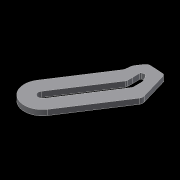
# Autodesk Inventor part: PelvisLinkLeft
Saved by Autodesk Inventor 2015 (Build 190159000, 159)
## iProperties
Created: 2014-12-04
Part Number: PelvisLinkLeft
Material: Generic
Document SubType Name: Modeling
Designer: Val
Density: 1 g/cm^3
Appearance: Default
Mass: 6.30084 g
Surface Area: 44.3973 cm^2
Volume: 6.30084 cm^3
Author: Val
Autodesk Inventor part; units mm, degrees
ref_plane "YZ Plane" through (0, 0, 0) normal (1, 0, 0) x (0, 1, 0)
ref_plane "XZ Plane" through (0, 0, 0) normal (0, 1, 0) x (-1, 0, 0)
ref_plane "XY Plane" through (0, 0, 0) normal (0, 0, 1) x (1, 0, 0)
sketch "Body" plane through (0, 0, 0) normal (0, 0, 1) x (1, 0, 0)
  line L0 (28.8487, 38.4543) -> (2.7256, -1.7701)
  line L1 (22.3487, 40.3798) -> (-2.7256, 1.7701)
  line L2 (22.3487, 40.3798) -> (22.3487, 45.0293)
  line L3 (28.8487, 38.4543) -> (28.8487, 45.9543)
  line L4 (32.4946, 58.4071) -> (39.19, 35.3599)
  line L5 (19.5232, 59.2689) -> (32.4946, 58.4071)
  line L6 (14.1445, 46.7648) -> (14.7577, 52.2305)
  line L7 (22.3487, 45.0293) -> (20.7935, 50.3829) construction
  line L8 (28.8487, 45.9543) -> (27.0354, 52.1963) construction
  arc A0 (-11.4127, 7.4118) -> (11.4127, -7.4118) centre (0, 0) ccw
  line L9 (-11.4127, 7.4118) -> (14.1445, 46.7648)
  line L10 (11.4127, -7.4118) -> (39.19, 35.3599)
  circle A1 centre (0, 0) radius 3.25
  line L11 (25.5987, 39.4171) -> (0, 0) construction
  line L12 (25.5987, 39.4171) -> (25.5987, 45.4918) construction
  line L13 (25.5987, 45.4918) -> (24.7618, 48.3727) construction
  line L14 (19.5232, 59.2689) -> (14.7577, 52.2305)
  line L15 (-30.4273, 0) -> (50.7929, 0) construction
  line L16 (20.7935, 50.3829) -> (22.2339, 50.8014) construction
  line L17 (22.3487, 45.0293) -> (22.2339, 50.8014)
  line L18 (28.8487, 45.9543) -> (25.595, 51.7778)
  line L19 (22.2339, 50.8014) -> (25.595, 51.7778)
  line L20 (25.595, 51.7778) -> (27.0354, 52.1963) construction
  dimension "d37" = 6.5
  dimension "d38" = 130.8
  dimension "d45" = 3.25
  dimension "d46" = 3.25
  dimension "d47" = 3.25
  dimension "d48" = 3.25
  dimension "d49" = 3.25
  dimension "d50" = 3.25
  dimension "d51" = 47
  dimension "d52" = 7.5
  dimension "d54" = 123.001
  dimension "d56" = 130.8
  dimension "d57" = 24
  dimension "d58" = 13
  dimension "d59" = 8.5
  dimension "d60" = 5.5
  dimension "d61" = 110
  dimension "d62" = 120.3
  dimension "d63" = 51
  dimension "d64" = 153.4
  dimension "d74" = 6.5
  dimension "d75" = 1.5
  dimension "d76" = 1.5
  constraints: 40 end point, 6 parallel, 4 point on circle, 3 perpendicular, 2 centre point, 2 tangent, 1 coincident, 1 point on line, 1 vertical
  measures "d37" diameter of A1
  measures "d38" angle of L11 L13
  measures "d45" distance between parallel lines of L1 L11
  measures "d46" distance between parallel lines of L2 L12
  measures "d47" distance between parallel lines of L7 L13
  measures "d48" distance between parallel lines of L0 L11
  measures "d49" distance between parallel lines of L3 L12
  measures "d50" distance between parallel lines of L13 L8
  measures "d51" distance of L11.end L11.start
  measures "d52" distance of L0.start L3.end
  measures "d54" angle of L9 L15
  measures "d56" angle of L10 L4
  measures "d57" distance of L4.start L4.end
  measures "d58" distance of L5.start L4.start
  measures "d59" distance of L5.start L6.end
  measures "d60" distance of L6.start L6.end
  measures "d61" angle of L4 L5
  measures "d62" angle of L5 L14
  measures "d63" distance of L10.start L4.end
  measures "d64" angle of L6 L9
  measures "d74" distance of L3.end L8.end
  measures "d75" distance of L16.end L7.end
  measures "d76" distance of L8.end L18.end
extrude "BodyFeature" add sketch "Body" along normal blind 4
fillet "BodyFillet1Feature" radius 3.5 1 edges at (19.5232, 59.2689, 2)
fillet "BodyFillet2Feature" radius 5 1 edges at (14.7577, 52.2305, 2)
fillet "BodyFillet3Feature" radius 2 1 edges at (32.4946, 58.4071, 2)
fillet "BodyFillet4Feature" radius 4 1 edges at (39.19, 35.3599, 2)
fillet "BodyFillet5Feature" radius 5 1 edges at (14.1445, 46.7648, 2)
fillet "InsideFilletsFeature" radius 3 4 edges at (22.3487, 40.3798, 2) (22.3487, 45.0293, 2) (28.8487, 45.9543, 2) (28.8487, 38.4543, 2)
fillet "InsideFilletsSmallFeature" radius 1 2 edges at (22.2339, 50.8014, 2) (25.595, 51.7778, 2)
